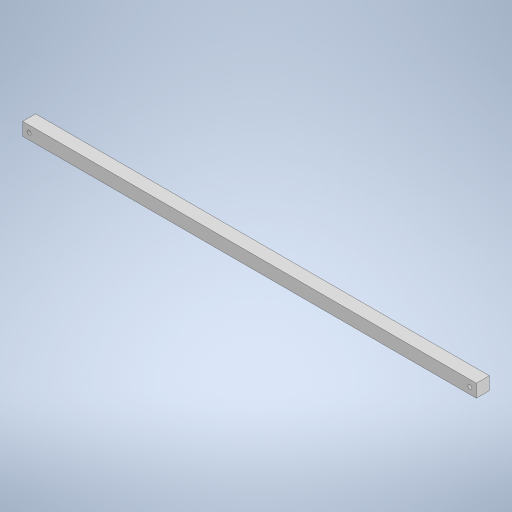
# Autodesk Inventor part: SokuYoko
Saved by Autodesk Inventor 2023 (Build 270158000, 158)
## iProperties
Created: 2022-10-24
Part Number: SokuYoko
Material: 一般
Document SubType Name: Modeling
Designer: banru
Density: 1 g/cm^3
Appearance: 既定
Author: banru
Autodesk Inventor part; units mm, degrees
ref_plane "YZ Plane" through (0, 0, 0) normal (1, 0, 0) x (0, 1, 0)
ref_plane "XZ Plane" through (0, 0, 0) normal (0, 1, 0) x (-1, 0, 0)
ref_plane "XY Plane" through (0, 0, 0) normal (0, 0, 1) x (1, 0, 0)
sketch "スケッチ1" plane through (0, 0, 0) normal (0, 1, 0) x (-1, 0, 0)
  line L0 (0, 0) -> (350, 0)
  line L1 (350, 0) -> (350, -10)
  line L2 (350, -10) -> (0, -10)
  line L3 (0, -10) -> (0, 0)
  dimension "d0" = 350
  dimension "d1" = 10
  constraints: 8 end point, 2 parallel, 1 horizontal, 1 perpendicular
  measures "d0" distance of L1.end L2.end
  measures "d1" distance of L0.end L1.end
extrude "押し出し1" add sketch "スケッチ1" along normal blind 10
sketch "スケッチ2" plane through (-350, 0, 0) normal (0, 0, 1) x (1, 0, 0)
  line L0 (350, 0) -> (350, 10) projected
  line L1 (0, 0) -> (0, 10) projected
  point P0 (345, 5)
  point P1 (5, 4.9593)
  point P2 (350, 5)
  point P3 (350, 5)
  point P4 (0, 5)
  dimension "d4" = 5
  dimension "d5" = 5
  constraints: 3 midpoint, 1 horizontal alignment
  measures "d4" distance of point (350, 5) point (345, 5)
  measures "d5" horizontal distance of point (5, 4.959) point (0, 5)
hole "穴1" at (-5, 5, 0) at (-345, 4.9593, 0) direction (0, 0, -1) diameter 3.1 end through all
